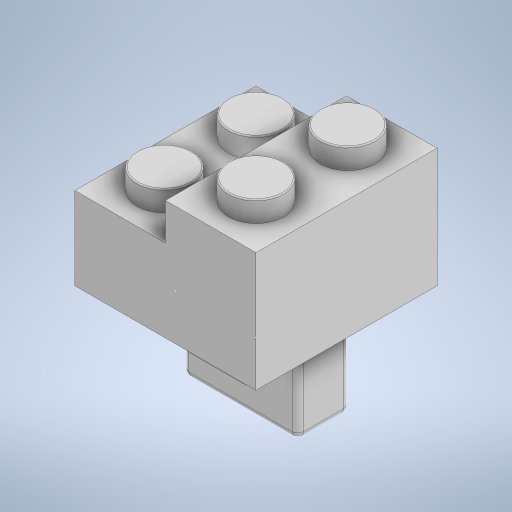
# Autodesk Inventor part: LEGO_hanging_brick
Saved by Autodesk Inventor 2024 (Build 280153000, 153)
## iProperties
Created: 2024-01-05
Part Number: LEGO_hanging_brick
Material: Generic
Document SubType Name: Modeling
Designer: kamil
Density: 1 g/cm^3
Appearance: Default
Author: kamil
Autodesk Inventor part; units mm, degrees
ref_plane "YZ Plane" through (0, 0, 0) normal (1, 0, 0) x (0, 1, 0)
ref_plane "XZ Plane" through (0, 0, 0) normal (0, 1, 0) x (-1, 0, 0)
ref_plane "XY Plane" through (0, 0, 0) normal (0, 0, 1) x (1, 0, 0)
sketch "Sketch1" plane through (0, 0, 0) normal (0, 1, 0) x (-1, 0, 0)
  line L0 (0, 0) -> (15.8, 0)
  line L1 (15.8, 0) -> (15.8, -15.8)
  line L2 (15.8, -15.8) -> (0, -15.8)
  line L3 (0, -15.8) -> (0, 0)
  dimension "d0" = 15.8
  dimension "d1" = 15.8
  constraints: 8 end point, 2 parallel, 1 horizontal, 1 perpendicular
  measures "d0" distance of L1.end L2.end
  measures "d1" distance of L0.end L1.end
extrude "Extrusion1" add sketch "Sketch1" along normal blind 3.2
sketch "Sketch2" plane through (0, 3.2, 0) normal (0, 1, 0) x (1, 0, 0)
  line L0 (-15.8, 0) -> (0, 0) projected
  line L1 (0, 15.8) -> (-15.8, 15.8) projected
  line L2 (0, 0) -> (-7.9, 0)
  line L3 (-7.9, 0) -> (-7.9, 15.8)
  line L4 (-7.9, 15.8) -> (0, 15.8)
  line L5 (0, 15.8) -> (0, 0)
  dimension "d4" = 7.9
  constraints: 8 end point, 2 parallel, 1 horizontal, 1 midpoint, 1 perpendicular
  measures "d4" distance of L3.end L4.end
extrude "Extrusion2" add sketch "Sketch2" along normal blind 3.2
sketch "Sketch3" plane through (0, 6.4, 0) normal (0, 1, 0) x (1, 0, 0)
  circle A0 centre (-3.9, 11.9) radius 2.4
  line L0 (0, 15.8) -> (-7.9, 15.8) projected
  line L1 (0, 0) -> (0, 15.8) projected
  line L2 (0, 7.9) -> (-7.9, 7.9) construction
  line L3 (-7.9, 15.8) -> (-7.9, 0) construction
  circle A1 centre (-3.9, 3.9) radius 2.4
  dimension "d7" = 4.8
  dimension "d8" = 3.9
  dimension "d9" = 3.9
  dimension "d10" = 8
  constraints: 2 centre point, 2 end point, 2 midpoint, 1 symmetric about line, 1 other
  measures "d7" diameter of A0
  measures "d8" distance from line of L0 A0.centre
  measures "d9" distance from line of L1 A0.centre
  measures "d10" distance of A1.centre A0.centre
sketch "Sketch4" plane through (0, 3.2, 0) normal (0, 1, 0) x (1, 0, 0)
  circle A0 centre (-11.9, 11.9) radius 2.4
  line L0 (-7.9, 15.8) -> (-15.8, 15.8) projected
  line L1 (-15.8, 15.8) -> (-15.8, 0) projected
  line L2 (-7.9, 15.8) -> (-7.9, 0) construction
  line L3 (-7.9, 7.9) -> (-15.8, 7.9) construction
  circle A1 centre (-11.9, 3.9) radius 2.4
  point P0 (0, 0)
  dimension "d11" = 4.8
  dimension "d12" = 3.9
  dimension "d13" = 3.9
  constraints: 2 centre point, 2 end point, 2 midpoint, 1 symmetric about line, 1 other
  measures "d11" diameter of A0
  measures "d12" distance from line of L0 A0.centre
  measures "d13" distance from line of L1 A0.centre
extrude "Extrusion3" add sketch "Sketch4" along normal blind 1.8
extrude "Extrusion4" add sketch "Sketch3" along normal blind 1.8
sketch "Sketch5" plane through (0, 0, 0) normal (0, -1, 0) x (1, 0, 0)
  point P0 (0, 0)
sketch "Sketch6" plane through (0, 0, 0) normal (0, -1, 0) x (1, 0, 0)
  point P0 (0, 0)
sketch "Sketch7" plane through (0, 0, 0) normal (0, -1, 0) x (1, 0, 0)
  line L0 (-7.9, 0) -> (0, 0) projected
  line L1 (0, 0) -> (-15.8, 0)
  line L2 (-15.8, 0) -> (-15.8, -15.8)
  line L3 (-15.8, -15.8) -> (0, -15.8)
  line L4 (0, -15.8) -> (0, 0)
  constraints: 8 end point, 2 parallel, 1 horizontal, 1 perpendicular
extrude "Extrusion5" add sketch "Sketch7" along normal blind 4
sketch "Sketch8" plane through (0, -4, 0) normal (0, -1, 0) x (1, 0, 0)
  line L0 (-2, -5.65) -> (-7, -5.65)
  line L1 (-7, -5.65) -> (-7, -10.15)
  line L2 (-7, -10.15) -> (-2, -10.15)
  line L3 (-2, -10.15) -> (-2, -5.65)
  line L4 (0, 0) -> (0, -15.8) construction
  line L5 (0, -7.9) -> (-15.8, -7.9) construction
  line L6 (-15.8, -15.8) -> (-15.8, 0) construction
  point P0 (-2, -7.9)
  dimension "d20" = 4.5
  dimension "d21" = 5
  dimension "d22" = 0
  dimension "d24" = 7
  constraints: 10 end point, 3 midpoint, 2 parallel, 1 horizontal, 1 perpendicular
  measures "d20" distance of L1.end L0.end
  measures "d21" distance of L1.end L2.end
  measures "d22" distance from line of L5 point (-2, -7.9)
  measures "d24" distance between parallel lines of L4 L1
extrude "Extrusion6" add sketch "Sketch8" along normal blind 7.7
sketch "Sketch9" plane through (-7, -4, -10.15) normal (-1, 0, 0) x (0, 0, 1)
  point P0 (10.15, 4)
sketch "Sketch10" plane through (-7, -4, -10.15) normal (-1, 0, 0) x (0, 0, 1)
  line L0 (4.5, 0) -> (4.5, -7.7) projected
  line L1 (0, 0) -> (0, -7.7) projected
  line L2 (4.5, -7.7) -> (0, -7.7)
  line L3 (0, -7.7) -> (0, -5.2)
  line L4 (0, -5.2) -> (4.5, -5.2)
  line L5 (4.5, -5.2) -> (4.5, -7.7)
  point P0 (10.15, 4)
  point P1 (0, -7.7)
  point P2 (4.5, -5.2)
  dimension "d27" = 2.5
  constraints: 8 end point, 2 parallel, 1 horizontal, 1 perpendicular, 1 point on line
  measures "d27" distance of L2.end L3.end
extrude "Extrusion7" add sketch "Sketch10" along normal blind 5
fillet "Fillet1" radius 0.1 4 edges at (-6.3, 8.2, -3.9) (-14.3, 5, -3.9) (-14.3, 5, -11.9) (-6.3, 8.2, -11.9)
fillet "Fillet2" radius 0.5 13 edges at (-2, -7.85, -5.65) (-2, -7.85, -10.15) (-7, -11.7, -5.65) (-7, -11.7, -10.15) (-12, -11.7, -7.9) (-12, -10.45, -10.15) (-12, -10.45, -5.65) (-12, -9.2, -7.9) (-9.5, -9.2, -5.65) (-9.5, -9.2, -10.15) (-7, -6.6, -10.15) (-7, -6.6, -5.65) (-2, -11.7, -7.9)
body "Solid1"
